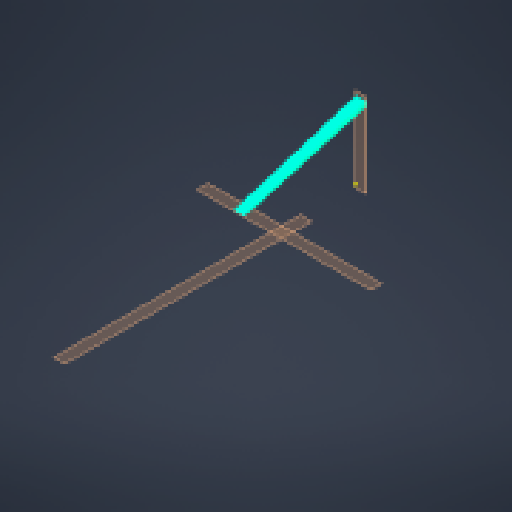
# Autodesk Inventor part: UpperEarDiagonal
Saved by Autodesk Inventor 2027 (Build 310192000, 192)
## iProperties
Created: 2026-08-07
Part Number: UpperEarDiagonal
Material: Generic
Document SubType Name: Modeling
Designer: lucas
Density: 1 g/cm^3
Appearance: Default
Author: lucas
Autodesk Inventor part; units mm, degrees
ref_plane "YZ Plane" through (0, 0, 0) normal (1, 0, 0) x (0, 1, 0)
ref_plane "XZ Plane" through (0, 0, 0) normal (0, 1, 0) x (-1, 0, 0)
ref_plane "XY Plane" through (0, 0, 0) normal (0, 0, 1) x (1, 0, 0)
ref_plane "Work Plane1" through (0, 0, 0) normal (0, 0, 1) x (1, 0, 0)
sketch "Sketch1" plane through (0, 0, 0) normal (0, 0, 1) x (1, 0, 0)
  line L0 (0, 762) -> (101.6, 762)
  line L1 (101.6, 762) -> (101.6, 711.2)
  line L2 (101.6, 711.2) -> (0, 711.2)
  line L3 (0, 711.2) -> (0, 762)
  point P0 (0, 0)
  dimension "d0" = 50.8
  dimension "d1" = 101.6
  constraints: 8 end point, 2 parallel, 1 horizontal, 1 perpendicular, 1 other
  measures "d0" distance of L0.end L1.end
  measures "d1" distance of L0.start L0.end
ref_plane "Work Plane2" through (50.8, 0, 1778) normal (0, 1, 0) x (0, 0, 1)
sketch "Sketch2" plane through (50.8, 0, 1778) normal (0, 1, 0) x (0, 0, 1)
  point P0 (-1778, -50.8)
ref_plane "Work Plane3" through (508, 379.808, 1169.3484) normal (0, 1, -0.0012) x (0, 0.0012, 1)
sketch "Sketch3" plane through (508, 379.808, 1169.3484) normal (0, 1, -0.0012) x (0, 0.0012, 1)
  line L0 (-509.4, -406.4) -> (1725.7984, -406.4) projected
  line L1 (-50.6969, 787.4) -> (-50.6969, -787.4) projected
  line L2 (50.6969, -787.4) -> (50.6969, 787.4) projected
  line L3 (1725.7984, -508) -> (-509.4, -508) projected
  line L4 (50.6969, -406.4) -> (-0.1031, -406.4)
  line L5 (-0.1031, -406.4) -> (-0.1031, -508)
  line L6 (-0.1031, -508) -> (50.6969, -508)
  line L7 (50.6969, -508) -> (50.6969, -406.4)
  point P0 (-1169.7996, -508)
  dimension "d2" = 50.8
  constraints: 8 end point, 3 point on line, 2 parallel, 1 horizontal, 1 perpendicular
  measures "d2" distance between parallel lines of L2 L5
loft "Loft1" add profiles "Sketch3", "Sketch1" contours L0 L2 L3 L5 / all
body "Solid1"
